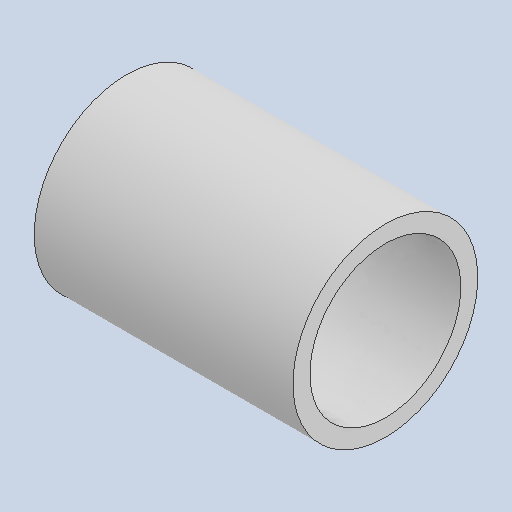
# Autodesk Inventor part: belt side spacer
Saved by Autodesk Inventor 2023 (Build 270158000, 158)
## iProperties
Created: 2022-09-05
Part Number: belt side spacer
Material: Generic
Document SubType Name: Modeling
Designer: deli
Density: 1 g/cm^3
Appearance: Default
Author: deli
Autodesk Inventor part; units mm, degrees
ref_plane "YZ Plane" through (0, 0, 0) normal (1, 0, 0) x (0, 1, 0)
ref_plane "XZ Plane" through (0, 0, 0) normal (0, 1, 0) x (-1, 0, 0)
ref_plane "XY Plane" through (0, 0, 0) normal (0, 0, 1) x (1, 0, 0)
sketch "Sketch1" plane through (0, 0, 0) normal (1, 0, 0) x (0, 1, 0)
  circle A0 centre (-71.3061, 55.1031) radius 7.5
  circle A1 centre (-71.3061, 55.1031) radius 6.125
  point P0 (0, 0)
  dimension "d0" = 15
  dimension "d1" = 12.25
  constraints: 2 centre point, 1 coincident
  measures "d0" diameter of A0
  measures "d1" diameter of A1
extrude "Extrusion1" add sketch "Sketch1" along normal blind 21
body "Solid1"
